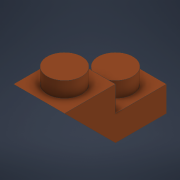
# Autodesk Inventor part: 110033226_ipt_11_樓梯支架
Saved by Autodesk Inventor 2022 (Build 260153000, 153)
## iProperties
Created: 2022-06-22
Part Number: 110033226_ipt_11_樓梯支架
Material: 一般
Document SubType Name: Modeling
Designer: User
Density: 1 g/cm^3
Appearance: 預設
Author: User
Autodesk Inventor part; units mm, degrees
ref_plane "YZ Plane" through (0, 0, 0) normal (1, 0, 0) x (0, 1, 0)
ref_plane "XZ Plane" through (0, 0, 0) normal (0, 1, 0) x (-1, 0, 0)
ref_plane "XY Plane" through (0, 0, 0) normal (0, 0, 1) x (1, 0, 0)
sketch "草圖1" plane through (0, 0, 0) normal (0, 1, 0) x (-1, 0, 0)
  line L0 (2.5, 5) -> (-2.5, 5)
  line L1 (-2.5, 5) -> (-2.5, -5)
  line L2 (-2.5, -5) -> (2.5, -5)
  line L3 (2.5, -5) -> (2.5, 5)
  circle A0 centre (0, 2.5) radius 1.7
  circle A1 centre (0, -2.5) radius 1.7
  line L4 (2.5, 0) -> (-2.5, 0)
  point P0 (0, 0)
  point P1 (0, -5)
  dimension "d0" = 5
  dimension "d1" = 10
  dimension "d2" = 3.4
  dimension "d3" = 3.4
  dimension "d4" = 2.5
  dimension "d5" = 2.5
  dimension "d6" = 2.5
  dimension "d7" = 2.5
  constraints: 10 end point, 3 midpoint, 2 centre point, 2 parallel, 1 horizontal, 1 horizontal alignment, 1 perpendicular, 1 vertical alignment
  measures "d0" distance of L2.end L1.end
  measures "d1" distance of L1.end L0.end
  measures "d2" diameter of A0
  measures "d3" diameter of A1
  measures "d4" distance from line of L3 A0.centre
  measures "d5" distance from line of L0 A0.centre
  measures "d6" distance from line of L2 A1.centre
  measures "d7" distance from line of L1 A1.centre
extrude "擠出1" add sketch "草圖1" along normal blind 2.5 contours L3 L2 L1 L4 | A1
extrude "擠出2" cut sketch "草圖1" along normal blind 1.5 contours A1
sketch "草圖2" plane through (0, 2.5, 0) normal (0, 1, 0) x (1, 0, 0)
  circle A0 centre (0, 2.5) radius 1.7 projected
  point P0 (0, 0)
extrude "擠出3" add sketch "草圖2" along normal blind 1.5
sketch "草圖3" plane through (0, 0, 0) normal (1, 0, 0) x (0, 1, 0)
  line L0 (0, 5) -> (0, -5) projected
  line L1 (0, 0) -> (5, 5)
  line L2 (5, 5) -> (5, 0)
  line L3 (5, 0) -> (0, 0)
  dimension "d15" = 5
  dimension "d20" = 5
  constraints: 6 end point, 1 perpendicular, 1 vertical
  measures "d15" distance of L2.end L1.start
  measures "d20" horizontal distance of L1.start L1.end
extrude "擠出4" add sketch "草圖3" along normal mid plane 5
sketch "草圖4" plane through (-2.5, 5, 5) normal (0, 1, 0) x (1, 0, 0)
  circle A0 centre (2.5, 2.5) radius 1.7 projected
  point P0 (2.5, 5)
extrude "擠出5" add sketch "草圖4" along normal blind 1.5
